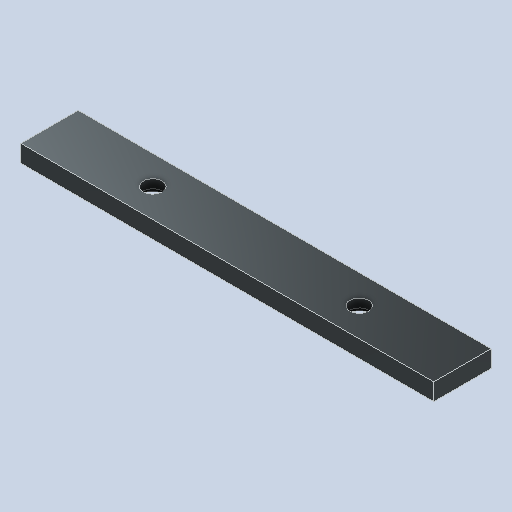
# Autodesk Inventor part: chapa_base
Saved by Autodesk Inventor 2022.2 (Build 262287010, 287A)
## iProperties
Created: 2022-03-09
Part Number: chapa_base
Material: Iron, Cast
Document SubType Name: Modeling
Designer: Korch
Density: 7.15 g/cm^3
Appearance: Iron Gray
Author: Korch
Autodesk Inventor part; units mm, degrees
ref_plane "YZ Plane" through (0, 0, 0) normal (1, 0, 0) x (0, 1, 0)
ref_plane "XZ Plane" through (0, 0, 0) normal (0, 1, 0) x (-1, 0, 0)
ref_plane "XY Plane" through (0, 0, 0) normal (0, 0, 1) x (1, 0, 0)
sketch "Sketch1" plane through (0, 0, 0) normal (0, 1, 0) x (-1, 0, 0)
  line L0 (0, 0) -> (-144, 0)
  line L1 (-144, 0) -> (-144, -20)
  line L2 (-144, -20) -> (0, -20)
  line L3 (0, -20) -> (0, 0)
  point P0 (-36, -10)
  point P1 (-108, -10)
  dimension "d0" = 144
  dimension "d1" = 20
  constraints: 8 end point, 2 parallel, 1 horizontal, 1 perpendicular
  measures "d0" distance of L2.end L1.end
  measures "d1" distance of L1.end L0.end
extrude "Extrusion1" add sketch "Sketch1" along normal blind 6
hole "Hole1" at (36, 0, -10) at (108, 0, -10) direction (0, 1, 0) diameter 6.6 end through all countersink diameter 12.6 countersink angle 90
body "Solid1"
